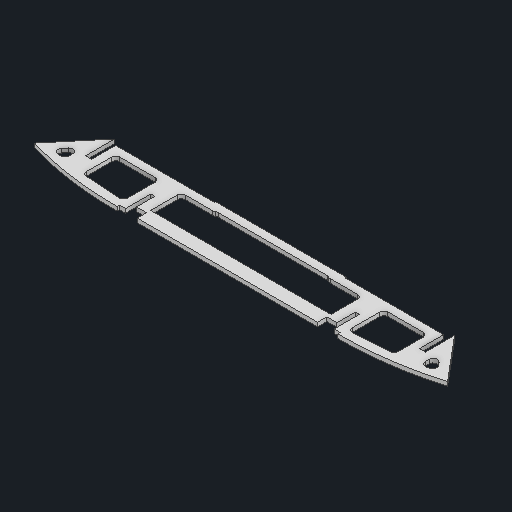
# Autodesk Inventor part: tail_2
Saved by Autodesk Inventor 2023 (Build 270158030, 158C)
## iProperties
Created: 2022-03-21
Part Number: tail_2
Material: Generic
Document SubType Name: Modeling
Designer: kardo
Density: 1 g/cm^3
Appearance: Default
Author: kardo
Autodesk Inventor part; units mm, degrees
ref_plane "YZ Plane" through (0, 0, 0) normal (1, 0, 0) x (0, 1, 0)
ref_plane "XZ Plane" through (0, 0, 0) normal (0, 1, 0) x (-1, 0, 0)
ref_plane "XY Plane" through (0, 0, 0) normal (0, 0, 1) x (1, 0, 0)
derived "parameters_frame.ipt"
derived "stencil_frame.ipt"
sketch "sk_joint_locations" plane through (81.12, 0, 0) normal (1, 0, 0) x (0, 1, 0)
  line L0 (0, 0) -> (122.4, 8.559) construction
  line L1 (36.465, 28.832) -> (112.2, 28.832) construction
  arc A0 (36.465, 28.832) -> (11.22, 28.376) centre (36.465, -670.197) ccw construction
  line L2 (-241.5001, 19.2432) -> (11.22, 28.376) construction
  line L3 (-345, 16.32) -> (-262.2001, 18.586) construction
  arc A1 (-262.2001, 18.586) -> (-241.5001, 19.2432) centre (-326.8578, 2381.2399) ccw construction
  line L4 (-95.1358, 3119.4657) -> (254.2444, -1876.9042) construction
  line L5 (-230.0001, 3089.1136) -> (-230.0001, -1866.0023) construction
  line L6 (-114.9999, 3089.1136) -> (-114.9999, -1866.0023) construction
  line L7 (-345, 3089.1136) -> (-345, -1866.0023) construction
  line L8 (0, 3089.1136) -> (0, -1866.0023) construction
  line L9 (516.4305, 45.5774) -> (-594.5903, 6.7797) construction
  line L10 (-657.7604, -27.3784) -> (621.8174, 62.0984) construction
  line L11 (193.4506, 30.2962) -> (193.1714, 38.2913) construction
  line L12 (201.1621, 36.7028) -> (201.7215, 28.7028) construction
  line L13 (0, 14.96) -> (121.9304, 15.2746) construction
  line L14 (-230.0001, 45.8702) -> (-230.0001, 19.6588) construction
  line L15 (-345, 37.4554) -> (-345, 16.32) construction
  line L16 (-114.9999, 51.0173) -> (-114.9999, 23.8147) construction
  line L17 (0, 52.89) -> (0, 27.9705) construction
  line L18 (119.462, 50.575) -> (119.9556, 43.5149) construction
  line L19 (120.4493, 36.4549) -> (119.9556, 43.5149) construction
  line L20 (120.4493, 36.4549) -> (120.943, 29.3948) construction
  line L21 (120.943, 29.3948) -> (121.4367, 22.3347) construction
  line L22 (121.4367, 22.3347) -> (121.9304, 15.2746) construction
  line L23 (0, 14.96) -> (0, 0) construction
  spline S0 degree 4 poles (-345, 37.4554) (-258.8682, 45.1562) (-172.5926, 49.7838) (-86.3161, 52.89) (0, 52.89) knots 0 0 0 0 0 1 1 1 1 1
  spline S1 degree 3 poles (0, 52.89) (92.8353, 52.89) (195.0311, 49.5089) (255, 36.448) knots 0 0 0 0 1 1 1 1
  spline S2 degree 2 poles (122.4, 8.559) (190.3044, 13.3074) (255, 36.448) knots 0 0 0 1 1 1
  line L24 (112.2, 37.536) -> (112.2, 28.832) construction
  line L25 (112.2, 35.548) -> (112.2, 30.82) construction
  point P0 (-95.1358, 3119.4657)
  point P1 (254.2444, -1876.9042)
  point P2 (193.311, 34.2938)
  point P3 (201.4418, 32.7028)
  point P4 (134.9575, 11.3411)
  point P5 (-345, 26.8877)
  point P6 (-230.0001, 32.7645)
  point P7 (-114.9999, 37.416)
  point P8 (0, 40.4303)
  point P9 (112.2, 33.184)
sketch "sk_cowl_joint_locations" plane through (54.6, 0, 0) normal (1, 0, 0) x (0, 1, 0)
  line L0 (-345, 16.32) -> (-262.2001, 18.586) construction
  arc A0 (-262.2001, 18.586) -> (-241.5001, 19.2432) centre (-326.8578, 2381.2399) ccw construction
  line L1 (-241.5001, 19.2432) -> (11.22, 28.376) construction
  arc A1 (36.465, 28.832) -> (11.22, 28.376) centre (36.465, -670.197) ccw construction
  line L2 (36.465, 28.832) -> (112.2, 28.832) construction
  line L3 (94.8, 30.032) -> (36.465, 30.032) construction
  arc A2 (36.465, 30.032) -> (11.1767, 29.5752) centre (36.465, -670.197) ccw construction
  line L4 (11.1767, 29.5752) -> (-241.5434, 20.4424) construction
  arc A3 (-262.2329, 19.7855) -> (-241.5434, 20.4424) centre (-326.8578, 2381.2399) ccw construction
  line L5 (-262.2329, 19.7855) -> (-345, 17.5204) construction
  line L6 (-230.0001, 3089.1136) -> (-230.0001, -1866.0023) construction
  line L7 (-114.9999, 3089.1136) -> (-114.9999, -1866.0023) construction
  line L8 (-345, 3089.1136) -> (-345, -1866.0023) construction
  line L9 (0, 3089.1136) -> (0, -1866.0023) construction
  line L10 (-230.0001, 45.0685) -> (-230.0001, 20.8596) construction
  line L11 (-114.9999, 49.9659) -> (-114.9999, 25.0155) construction
  line L12 (-345, 17.5204) -> (-345, 17.5204)
  line L13 (-345, 17.5204) -> (-345, 36.9221) construction
  line L14 (-869.78, 3004.1953) -> (348.339, -1881.413) construction
  line L15 (-344.7623, 36.9221) -> (-345, 39.712) construction
  line L16 (0, 51.6) -> (0, 29.1713) construction
  spline S0 degree 2 poles (-345, 39.712) (-172.656, 54.3934) (0, 54.4) knots 0 0 0 1 1 1
  spline S1 degree 3 poles (0, 54.4) (37.026, 54.4) (80.784, 47.9917) (112.2, 37.536) knots 1 1 1 1 2 2 2 2
  spline S2 degree 3 poles (111.3158, 34.8793) (106.1488, 36.5989) (96.4909, 39.4217) (84.5445, 42.2265) (75.2974, 44.1359) (69.0059, 45.3094) (61.0256, 46.6466) (54.5653, 47.6105) (46.4371, 48.6777) (39.9092, 49.4192) (31.7597, 50.2005) (25.2653, 50.7072) (17.2211, 51.1873) (9.2717, 51.5118) (3.0586, 51.6) (0, 51.6) knots 1 1 1 1 1.166667 1.291667 1.333333 1.416667 1.458333 1.541667 1.583333 1.666667 1.708333 1.791667 1.833333 1.916667 2 2 2 2
  spline S3 degree 3 poles (0, 51.6) (-19.1708, 51.5993) (-52.7146, 51.3604) (-91.0402, 50.6121) (-119.7801, 49.8472) (-138.9379, 49.2354) (-162.8824, 48.3434) (-182.0358, 47.528) (-205.975, 46.3814) (-225.1241, 45.3623) (-249.0578, 43.9611) (-268.2026, 42.7383) (-292.131, 41.0825) (-316.0566, 39.2994) (-335.1942, 37.7372) (-344.7623, 36.9221) knots 0 0 0 0 0.166667 0.291667 0.333333 0.416667 0.458333 0.541666 0.583333 0.666666 0.708333 0.791666 0.833333 0.916666 1 1 1 1
  line L17 (-136.2088, 45.4676) -> (-130.9657, 24.4385) construction
  line L18 (-128.3953, 30.6635) -> (-132.2764, 29.6958) construction
  line L19 (-131.0168, 41.178) -> (-134.898, 40.2103) construction
  line L20 (-136.2088, 45.4676) -> (-132.3276, 46.4353) construction
  line L21 (-130.9657, 24.4385) -> (-127.0845, 25.4062) construction
  line L22 (-132.3276, 46.4353) -> (-132.5171, 52.2322) construction
  point P0 (0, 0)
  point P1 (-345, 27.2213)
  point P2 (-230.0001, 32.964)
  point P3 (-114.9999, 37.4907)
  point P4 (0, 40.3857)
  point P5 (-869.78, 3004.1953)
  point P6 (348.339, -1881.413)
  point P7 (-85.2629, 50.788)
  point P8 (0, 40.3857)
sketch "sk_tail_2_base" plane through (0, -230.0001, 0) normal (0, 1, 0) x (-1, 0, 0)
  spline S0 degree 2 poles (-54.6, 47.873) (-109.1649, 47.873) (-156, 15.1373) knots 0 0 0 1 1 1 construction
  line L0 (0, 47.873) -> (-54.6, 47.873) construction
  line L1 (890.7976, -1145.3209) -> (-1641.4492, 1872.4932) construction
  line L2 (0, -1866.0023) -> (0, 3089.1136) construction
  line L3 (0, 20.2827) -> (-32.32, 20.2827)
  line L4 (-32.32, 20.2827) -> (-32.32, 20.8588)
  line L5 (-32.32, 20.8588) -> (-81.12, 20.8588)
  line L6 (-81.12, 20.8588) -> (-81.12, 32.7645)
  line L7 (-81.12, 32.7645) -> (-84.12, 32.7645)
  line L8 (-84.12, 32.7645) -> (-84.12, 18.4075)
  line L9 (-84.12, 18.4075) -> (-102.2161, 39.9735)
  line L10 (0, 46.673) -> (-54.6, 46.673)
  line L11 (0, 46.673) -> (0, 20.2827)
  spline S1 degree 5 poles (-54.6, 46.673) (-65.2219, 46.6728) (-75.8434, 45.8932) (-86.3898, 44.2756) (-107.3821, 39.2832) (-127.3181, 31.0175) (-137.0542, 26.0451) (-146.3873, 20.3921) (-155.3125, 14.1538) knots 0 0 0 0 0 0 0.493789 0.493789 0.493789 1 1 1 1 1 1
  point P0 (0, 0)
  point P1 (-34.32, 19.6588)
  point P2 (-34.32, 19.0827)
  dimension "d3" = 1.2
  dimension "d4" = 1.2
  dimension "d5" = 1.2
  dimension "d6" = 2
  dimension "d7" = 3
  dimension "d8" = 1.2
  constraints: 18 end point, 5 parallel, 4 perpendicular, 2 point on line, 1 coincident, 4 other
  measures "d4" distance from line of L3 point (-34.32, 19.083)
  measures "d5" distance from line of L5 point (-34.32, 19.659)
  measures "d6" distance from line of point (-34.32, 19.659) L4
  measures "d7" distance of L6.end L7.end
  measures "d8" distance between parallel lines of L1 L9
extrude "thicken" add sketch "sk_tail_2_base" along normal blind 2
sketch "sk_cut_joint" plane through (0, -230.0001, 0) normal (0, 1, 0) x (-1, 0, 0)
  line L0 (0, 47.873) -> (-54.6, 47.873) projected
  line L1 (-54.6, -1866.0023) -> (-54.6, 3089.1136) construction
  line L2 (-49.6, 47.873) -> (-49.6, 32.964)
  line L3 (-49.6, 32.964) -> (-51.6, 32.964)
  line L4 (-51.6, 32.964) -> (-51.6, 47.873)
  point P0 (0, 0)
  point P1 (-54.6, 32.964)
  dimension "d11" = 5
  dimension "d12" = 2
  constraints: 6 end point, 3 parallel, 3 point on line
  measures "d11" distance between parallel lines of L1 L2
  measures "d12" distance between parallel lines of L2 L4
extrude "cut_joint" cut sketch "sk_cut_joint" along normal through all both and the other way through all
sketch "sk_cut_liner" plane through (0, -230.0001, 0) normal (0, 1, 0) x (-1, 0, 0)
  line L0 (0, 47.873) -> (-54.6, 47.873) projected
  line L1 (-54.6, -1866.0023) -> (-54.6, 3089.1136) projected
  line L2 (-44.6, 47.873) -> (-44.6, 42.073)
  line L3 (-44.6, 42.073) -> (-49.6, 42.073)
  line L4 (-49.6, 42.073) -> (-49.6, 45.473)
  line L5 (-49.6, 45.473) -> (-54.6, 45.473)
  point P0 (0, 0)
  dimension "d14" = 2.4
  dimension "d15" = 5
  dimension "d17" = 5
  dimension "d40" = 5.8
  constraints: 8 end point, 4 parallel, 2 point on line
  measures "d14" distance between parallel lines of L0 L5
  measures "d15" distance between parallel lines of L1 L4
  measures "d17" distance between parallel lines of L2 L4
  measures "d40" distance of L2.start L2.end
extrude "cut_liner" cut sketch "sk_cut_liner" along normal through all both and the other way through all
sketch "sk_cut_weight" plane through (0, -230.0001, 0) normal (0, 1, 0) x (-1, 0, 0)
  line L0 (-44.6, 47.873) -> (-44.6, 42.073) construction
  line L1 (-44.6, 42.073) -> (-49.6, 42.073) construction
  line L2 (-49.6, 42.073) -> (-49.6, 45.473) projected
  line L3 (-32.32, 20.8588) -> (-81.12, 20.8588) construction
  line L4 (-32.32, 20.2827) -> (-32.32, 20.8588) construction
  line L5 (0, 20.2827) -> (-32.32, 20.2827) construction
  line L6 (-81.12, 20.8588) -> (-81.12, 32.7645) construction
  line L7 (-84.12, 32.7645) -> (-84.12, 18.4075) construction
  spline S0 degree 3 poles (-54.6, 46.673) (-57.6114, 46.673) (-63.5979, 46.5224) (-70.9907, 45.958) (-78.3162, 45.1115) (-84.1227, 44.2086) (-91.3139, 42.7979) (-97.0135, 41.4437) (-104.0715, 39.4688) (-109.6649, 37.6631) (-116.5906, 35.1235) (-122.0784, 32.8659) (-130.2315, 29.1403) (-140.9623, 23.5695) (-150.1385, 17.7702) (-155.3125, 14.1538) knots 0 0 0 0 0.083333 0.166667 0.208333 0.291667 0.333333 0.416667 0.458333 0.541667 0.583333 0.666667 0.708333 0.833333 1 1 1 1 construction
  line L8 (-84.12, 18.4075) -> (-102.2161, 39.9735) construction
  line L9 (0, -1866.0023) -> (0, 3089.1136) projected
  line L10 (-88.12, 29.3974) -> (-88.12, 39.419)
  line L11 (-88.12, 39.419) -> (-95.4077, 38.0825)
  line L12 (-95.4077, 38.0825) -> (-88.12, 29.3974)
  line L13 (-88.12, 39.419) -> (-88.12, 43.419) construction
  line L14 (-95.4077, 38.0825) -> (-97.9788, 41.1467) construction
  line L15 (0, 40.073) -> (-44.6, 40.073)
  line L16 (-44.6, 40.073) -> (-44.6, 24.8588)
  line L17 (-44.6, 24.8588) -> (-28.32, 24.8588)
  line L18 (-28.32, 24.8588) -> (-28.32, 24.2827)
  line L19 (-28.32, 24.2827) -> (0, 24.2827)
  line L20 (-55.6, 42.673) -> (-77.12, 41.2)
  line L21 (-77.12, 41.2) -> (-77.12, 24.8588)
  line L22 (-77.12, 24.8588) -> (-55.6, 24.8588)
  line L23 (-55.6, 24.8588) -> (-55.6, 42.673)
  line L24 (-49.6, 42.073) -> (-49.6, 20.8588) construction
  line L25 (-49.6, 42.073) -> (-51.6, 42.073) construction
  line L26 (-51.6, 42.073) -> (-51.6, 20.8588) construction
  line L27 (-77.12, 41.2) -> (-77.3931, 45.1907) construction
  point P0 (0, 0)
  dimension "d22" = 2
  dimension "d23" = 4
  dimension "d24" = 4
  dimension "d25" = 4
  dimension "d26" = 4
  dimension "d28" = 4
  dimension "d29" = 4
  dimension "d30" = 4
  dimension "d31" = 4
  dimension "d32" = 4
  dimension "d33" = 4
  dimension "d34" = 4
  dimension "d35" = 2
  dimension "d39" = 4
  constraints: 36 end point, 11 parallel, 4 collinear, 4 point on line, 2 perpendicular, 3 other
  measures "d22" distance between parallel lines of L24 L26
  measures "d23" distance between parallel lines of L23 L26
  measures "d24" distance between parallel lines of L3 L22
  measures "d25" distance between parallel lines of L6 L21
  measures "d26" distance of L20.end L27.end
  measures "d28" distance between parallel lines of L7 L10
  measures "d29" distance between parallel lines of L8 L12
  measures "d30" distance of L10.end L13.end
  measures "d31" distance of L11.end L14.end
  measures "d32" distance between parallel lines of L5 L19
  measures "d33" distance between parallel lines of L4 L18
  measures "d34" distance between parallel lines of L3 L17
  measures "d35" distance between parallel lines of L1 L15
  measures "d39" vertical distance of L20.start point (-54.6, 46.673)
extrude "cut_weight" cut sketch "sk_cut_weight" along normal through all both and the other way through all
fillet "rounding" radius 2 10 edges at (28.32, -229.0001, 24.8588) (28.32, -229.0001, 24.2827) (44.6, -229.0001, 24.8588) (77.12, -229.0001, 41.2) (95.4077, -229.0001, 38.0825) (77.12, -229.0001, 24.8588) (88.12, -229.0001, 29.3974) (55.6, -229.0001, 24.8588) (55.6, -229.0001, 42.673) (88.12, -229.0001, 39.419)
mirror "mirror" about plane through (0, 0, 0) normal (1, 0, 0)
equation "\"d3\" = shell_thickness"
equation "\"d4\" = shell_thickness"
equation "\"d5\" = shell_thickness"
equation "\"d6\" = bulkhead_thickness"
equation "\"d7\" = stringer_thickness"
equation "\"d8\" = shell_thickness"
equation "\"d9\" = bulkhead_thickness"
equation "\"d11\" = cowl_liner_width"
equation "\"d12\" = bulkhead_thickness"
equation "\"d14\" = shell_thickness + cowl_liner_thickness"
equation "\"d15\" = cowl_liner_width"
equation "\"d17\" = cowl_sealing_width"
equation "\"d40\" = cowl_sealing_thickness + cowl_shell_thickness + cowl_liner_thickness"
equation "\"d22\" = bulkhead_thickness"
equation "\"d23\" = bulkhead_inset"
equation "\"d24\" = bulkhead_inset"
equation "\"d25\" = bulkhead_inset"
equation "\"d26\" = bulkhead_inset"
equation "\"d28\" = bulkhead_inset"
equation "\"d29\" = bulkhead_inset"
equation "\"d30\" = bulkhead_inset"
equation "\"d31\" = bulkhead_inset"
equation "\"d32\" = bulkhead_inset"
equation "\"d33\" = bulkhead_inset"
equation "\"d34\" = bulkhead_inset"
equation "\"d39\" = bulkhead_inset"
equation "\"d38\" = 0.5 * bulkhead_inset"
equation "\"shell_thickness\" = 1.2"
equation "\"stringer_thickness\" = 3"
equation "\"bulkhead_thickness\" = 2"
equation "\"cowl_liner_width\" = 5"
equation "\"cowl_liner_thickness\" = 1.2"
equation "\"cowl_sealing_width\" = 5"
equation "\"cowl_sealing_thickness\" = 3"
equation "\"cowl_shell_thickness\" = 1.6"
equation "\"bulkhead_inset\" = 4"
body "Solid1"
